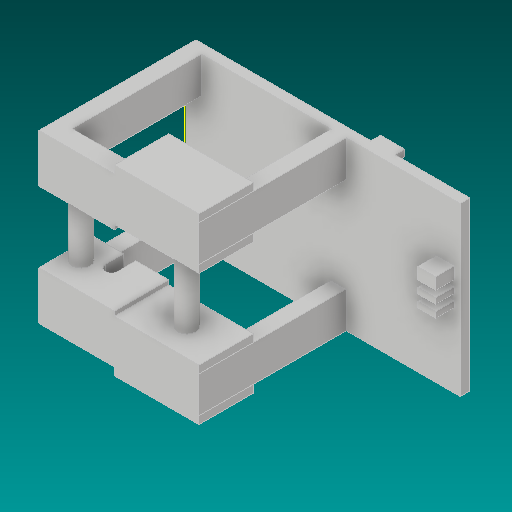
# Autodesk Inventor part: RC_Chassis
Saved by Autodesk Inventor 2019 (Build 230136000, 136)
## iProperties
Created: 2020-12-08
Part Number: RC_Chassis
Material: Generic
Document SubType Name: Modeling
Designer: Jason
Density: 1 g/cm^3
Appearance: Default
Mass: 177.89 g
Surface Area: 666.663 cm^2
Volume: 177.89 cm^3
Author: Jason
Autodesk Inventor part; units mm, degrees
ref_plane "YZ Plane" through (0, 0, 0) normal (1, 0, 0) x (0, 1, 0)
ref_plane "XZ Plane" through (0, 0, 0) normal (0, 1, 0) x (-1, 0, 0)
ref_plane "XY Plane" through (0, 0, 0) normal (0, 0, 1) x (1, 0, 0)
sketch "Sketch1" plane through (0, 0, 0) normal (0, 0, 1) x (1, 0, 0)
  line L0 (0, -53.3468) -> (0, -11.9835) projected
  line L1 (68.5887, -53.3468) -> (0, -53.3468) projected
  line L2 (68.5887, 0) -> (68.5887, -53.3468) projected
  line L3 (0, 0) -> (68.5887, 0) projected
  line L4 (0, -2.1686) -> (0, 0) projected
  line L5 (0, -11.9835) -> (0, -2.1686) projected
  circle A0 centre (15.2894, -50.7921) radius 1.5631 projected
  circle A1 centre (14.0269, -2.6176) radius 1.4996 projected
  line L6 (0, 0) -> (68.5887, 0)
  line L7 (68.5887, 0) -> (68.5887, -53.3468)
  line L8 (68.5887, -53.3468) -> (0, -53.3468)
  line L9 (0, -53.3468) -> (0, 0)
  circle A2 centre (14.0269, -2.6176) radius 1.4996
  circle A3 centre (15.2894, -50.7921) radius 1.5631
  constraints: 8 end point, 2 centre point, 2 coincident, 2 concentric, 2 parallel, 1 horizontal, 1 perpendicular
extrude "Extrusion1" add sketch "Sketch1" against normal blind 5.08 contours A0 | A1
ref_plane "Work Plane1" through (0, 0, 0) normal (0, 0, 1) x (1, 0, 0)
sketch "Sketch2" plane through (0, 0, 0) normal (0, 0, 1) x (1, 0, 0)
  line L0 (0, -53.3468) -> (0, -11.9835) projected
  line L1 (68.5887, 0) -> (68.5887, -53.3468) projected
  line L2 (0, -2.1686) -> (0, 0) projected
  line L3 (0, 0) -> (0, -53.3468)
  line L4 (68.5887, -53.3468) -> (68.5887, 0)
  line L5 (68.5887, -71.3254) -> (144.1005, -71.3254)
  line L6 (144.1005, -71.3254) -> (144.1005, 16.6007)
  line L7 (144.1005, 16.6007) -> (68.5887, 16.6007)
  line L8 (68.5887, 16.6007) -> (68.5887, -71.3254)
  line L9 (68.5887, 16.6007) -> (0, 16.6007)
  line L10 (0, 16.6007) -> (0, 0)
  line L11 (68.5887, -71.3254) -> (0, -71.3254)
  line L12 (0, -71.3254) -> (0, -53.3468)
  constraints: 20 end point, 4 perpendicular, 4 point on line, 3 parallel, 2 horizontal
extrude "Extrusion2" add sketch "Sketch2" along normal mid plane 5.08
sketch "Sketch3" plane through (0, 0, -2.54) normal (0, 0, -1) x (-1, 0, 0)
  line L0 (-125.7496, -4.4471) -> (-125.7496, -55.0115) projected
  line L1 (0, -71.3254) -> (-144.1005, -71.3254) projected
  line L2 (-125.7496, -38.1) -> (-133.2651, -38.1)
  line L3 (-133.2651, -38.1) -> (-133.2651, -17.4625)
  line L4 (-133.2651, -17.4625) -> (-125.7496, -17.4625)
  line L5 (-125.7496, -17.4625) -> (-125.7496, -38.1)
  line L6 (-125.7462, 13.1821) -> (-71.1251, 13.1821)
  line L7 (0, 16.6007) -> (-144.1005, 16.6007) projected
  line L8 (-92.075, 13.1821) -> (-104.775, 13.1821)
  line L9 (-104.775, 13.1821) -> (-104.775, 16.6007)
  line L10 (-104.775, 16.6007) -> (-92.075, 16.6007)
  line L11 (-92.075, 16.6007) -> (-92.075, 13.1821)
  line L12 (-80.6496, -69.3179) -> (-97.3996, -69.3179)
  line L13 (-144.1005, -71.3254) -> (0, -71.3254) projected
  line L14 (-97.3996, -69.3179) -> (-84.496, -69.3179)
  line L15 (-84.496, -69.3179) -> (-84.496, -71.3254)
  line L16 (-84.496, -71.3254) -> (-97.3996, -71.3254)
  line L17 (-97.3996, -71.3254) -> (-97.3996, -69.3179)
  point P0 (0, 0)
  point P1 (-68.5887, -71.3254)
  point P2 (-68.5887, 16.6007)
  constraints: 28 end point, 6 parallel, 4 point on line, 3 horizontal, 3 perpendicular
extrude "Extrusion3" add sketch "Sketch3" along normal blind 5.08
sketch "Sketch9" plane through (0, 0, 2.54) normal (0, 0, 1) x (1, 0, 0)
  line L0 (0, -71.3254) -> (7.9375, -71.3254)
  line L1 (7.9375, -71.3254) -> (7.9375, -52.2754)
  line L2 (7.9375, -52.2754) -> (0, -52.2754)
  line L3 (0, -52.2754) -> (0, -71.3254)
  line L4 (0, 16.6007) -> (7.9502, 16.6007)
  line L5 (7.9502, 16.6007) -> (7.9502, -2.4493)
  line L6 (7.9502, -2.4493) -> (0, -2.4493)
  line L7 (0, -2.4493) -> (0, 16.6007)
  line L8 (76.2, -71.3254) -> (84.1502, -71.3254)
  line L9 (84.1502, -71.3254) -> (84.1502, -52.2754)
  line L10 (84.1502, -52.2754) -> (76.2, -52.2754)
  line L11 (76.2, -52.2754) -> (76.2, -71.3254)
  line L12 (76.2, 16.6007) -> (84.1502, 16.6007)
  line L13 (84.1502, 16.6007) -> (84.1502, -2.4493)
  line L14 (84.1502, -2.4493) -> (76.2, -2.4493)
  line L15 (76.2, -2.4493) -> (76.2, 16.6007)
  line L16 (144.1005, 16.6007) -> (0, 16.6007) projected
  line L17 (0, -71.3254) -> (144.1005, -71.3254) projected
  point P0 (0, 0)
  dimension "d19" = 7.9502
  dimension "d20" = 19.05
  dimension "d21" = 7.9502
  dimension "d22" = 19.05
  dimension "d23" = 7.9502
  dimension "d24" = 19.05
  dimension "d41" = 19.05
  constraints: 32 end point, 8 parallel, 4 horizontal, 4 perpendicular, 2 collinear, 1 point on line
  measures "d19" distance of L5.end L6.end
  measures "d20" distance of L4.end L5.end
  measures "d21" distance of L10.end L9.end
  measures "d22" distance of L9.end L8.end
  measures "d23" distance of L13.end L14.end
  measures "d24" distance of L12.end L13.end
  measures "d41" distance of L0.end L1.end
extrude "Extrusion7" add sketch "Sketch9" along normal blind 67.945
sketch "Sketch10" plane through (0, 0, 2.54) normal (0, 0, 1) x (1, 0, 0)
  line L0 (141.2875, -13.0792) -> (131.7625, -13.0792)
  line L1 (131.7625, -13.0792) -> (131.7625, -19.4292)
  line L2 (131.7625, -19.4292) -> (141.2875, -19.4292)
  line L3 (141.2875, -19.4292) -> (141.2875, -13.0792)
  line L4 (141.2875, -22.6042) -> (131.7625, -22.6042)
  line L5 (131.7625, -22.6042) -> (131.7625, -25.7792)
  line L6 (131.7625, -25.7792) -> (141.2875, -25.7792)
  line L7 (141.2875, -25.7792) -> (141.2875, -22.6042)
  line L8 (141.2875, -28.9542) -> (131.7625, -28.9542)
  line L9 (131.7625, -28.9542) -> (131.7625, -32.1292)
  line L10 (131.7625, -32.1292) -> (141.2875, -32.1292)
  line L11 (141.2875, -32.1292) -> (141.2875, -28.9542)
  line L12 (144.1005, 16.6007) -> (84.1502, 16.6007) projected
  line L13 (84.1502, -71.3254) -> (144.1005, -71.3254) projected
  line L14 (90.4875, -27.3667) -> (109.5375, -27.3667)
  point P0 (0, 0)
  dimension "d30" = 3.175
  dimension "d31" = 3.175
  dimension "d32" = 3.175
  dimension "d33" = 3.175
  dimension "d39" = 6.35
  dimension "d70" = 43.9674
  constraints: 26 end point, 6 parallel, 4 horizontal, 3 perpendicular, 1 point on line, 1 other
  measures "d30" distance of L5.end L4.end
  measures "d31" distance of L9.end L8.end
  measures "d32" distance between parallel lines of L4 L2
  measures "d33" distance between parallel lines of L8 L6
  measures "d39" distance of L0.end L1.end
  measures "d70" distance between parallel lines of L14 L12
extrude "Extrusion8" add sketch "Sketch10" along normal blind 10.16
sketch "Sketch11" plane through (0, 0, 70.485) normal (0, 0, 1) x (1, 0, 0)
  line L0 (0, 16.6007) -> (84.1502, 16.6007)
  line L1 (84.1502, 16.6007) -> (84.1502, -2.4493)
  line L2 (84.1502, -2.4493) -> (0, -2.4493)
  line L3 (0, -2.4493) -> (0, 16.6007)
  line L4 (0, -71.3254) -> (7.9375, -71.3254) projected
  line L5 (0, -71.3254) -> (84.1502, -71.3254)
  line L6 (84.1502, -71.3254) -> (84.1502, -52.2754)
  line L7 (84.1502, -52.2754) -> (0, -52.2754)
  line L8 (0, -52.2754) -> (0, -71.3254)
  point P0 (0, 0)
  dimension "d44" = 19.05
  dimension "d45" = 19.05
  constraints: 16 end point, 4 parallel, 2 horizontal, 2 perpendicular, 1 point on line
  measures "d44" distance between parallel lines of L0 L2
  measures "d45" distance between parallel lines of L5 L7
extrude "Extrusion9" add sketch "Sketch11" along normal blind 9.525
sketch "Sketch12" plane through (0, 0, 70.485) normal (0, 0, -1) x (-1, 0, 0)
  line L0 (0, 16.6007) -> (-92.075, 16.6007) projected
  line L1 (-84.1375, 16.6007) -> (-39.6875, 16.6007)
  line L2 (-39.6875, 16.6007) -> (-39.6875, 20.6375)
  line L3 (-39.6875, 20.6375) -> (-84.1375, 20.6375)
  line L4 (-84.1375, 20.6375) -> (-84.1375, 16.6007)
  line L5 (-84.1375, -6.4861) -> (-39.6875, -6.4861)
  line L6 (-39.6875, -6.4861) -> (-39.6875, -2.4493)
  line L7 (-39.6875, -2.4493) -> (-84.1375, -2.4493)
  line L8 (-84.1375, -2.4493) -> (-84.1375, -6.4861)
  line L9 (-84.1375, -52.2754) -> (-39.6875, -52.2754)
  line L10 (-39.6875, -52.2754) -> (-39.6875, -48.2386)
  line L11 (-39.6875, -48.2386) -> (-84.1375, -48.2386)
  line L12 (-84.1375, -48.2386) -> (-84.1375, -52.2754)
  line L13 (-84.1375, -75.3622) -> (-39.6875, -75.3622)
  line L14 (-39.6875, -75.3622) -> (-39.6875, -71.3254)
  line L15 (-39.6875, -71.3254) -> (-84.1375, -71.3254)
  line L16 (-84.1375, -71.3254) -> (-84.1375, -75.3622)
  line L17 (0, -2.4493) -> (-84.1502, -2.4493) projected
  line L18 (-84.1502, -52.2754) -> (0, -52.2754) projected
  line L19 (0, -71.3254) -> (-84.1502, -71.3254) projected
  line L20 (0, -2.4493) -> (0, -52.2754) projected
  line L21 (-39.6875, -52.2754) -> (0, -52.2754)
  line L22 (0, -52.2754) -> (0, -45.9254)
  line L23 (0, -45.9254) -> (-39.6875, -45.9254)
  line L24 (-39.6875, -45.9254) -> (-39.6875, -52.2754)
  line L25 (-39.6875, -2.4493) -> (0, -2.4493)
  line L26 (0, -2.4493) -> (0, -8.7993)
  line L27 (0, -8.7993) -> (-39.6875, -8.7993)
  line L28 (-39.6875, -8.7993) -> (-39.6875, -2.4493)
  point P0 (0, 0)
  dimension "d46" = 4.0368
  dimension "d53" = 44.45
  dimension "d54" = 6.35
  dimension "d55" = 6.35
  constraints: 48 end point, 12 collinear, 12 parallel, 6 horizontal, 6 perpendicular, 3 point on line
  measures "d46" distance of L3.end L1.start
  measures "d53" distance of L2.end L3.end
  measures "d54" distance of L22.end L21.end
  measures "d55" distance of L25.end L26.end
extrude "Extrusion10" add sketch "Sketch12" along normal blind 19.05 and the other way blind 9.525
sketch "Sketch13" plane through (0, -45.9254, 51.435) normal (0, 1, 0) x (1, 0, 0)
  line L0 (19.1249, 12.586) -> (19.1249, -9.639) construction
  line L1 (15.9499, 12.586) -> (15.9499, -9.639)
  line L2 (22.2999, -9.639) -> (22.2999, 12.586)
  arc A0 (22.2999, 12.586) -> (15.9499, 12.586) centre (19.1249, 12.586) ccw
  arc A1 (15.9499, -9.639) -> (22.2999, -9.639) centre (19.1249, -9.639) ccw
  point P0 (0, 51.435)
  point P1 (19.1249, 1.4735)
  constraints: 8 end point, 4 point on circle, 4 tangent, 2 centre point, 1 midpoint, 1 parallel, 1 vertical
extrude "Extrusion11" cut sketch "Sketch13" against normal blind 8.255
sketch "Sketch14" plane through (0, -8.7993, 51.435) normal (0, -1, 0) x (1, 0, 0)
  line L0 (19.1249, 12.586) -> (19.1249, -9.639) construction
  line L1 (15.9499, 12.586) -> (15.9499, -9.639)
  line L2 (22.2999, -9.639) -> (22.2999, 12.586)
  arc A0 (22.2999, 12.586) -> (15.9499, 12.586) centre (19.1249, 12.586) ccw
  arc A1 (15.9499, -9.639) -> (22.2999, -9.639) centre (19.1249, -9.639) ccw
  point P0 (0, 51.435)
  point P1 (19.1249, 1.4735)
  constraints: 8 end point, 4 point on circle, 4 tangent, 2 centre point, 1 midpoint, 1 parallel, 1 vertical
extrude "Extrusion12" cut sketch "Sketch14" against normal blind 8.255
sketch "Sketch15" plane through (39.6875, -6.4861, 51.435) normal (0, -1, 0) x (1, 0, 0)
  circle A0 centre (23.8125, 14.2875) radius 4.7625
  line L0 (-31.7373, -48.895) -> (-31.7373, 19.05) projected
  circle A1 centre (-31.7373, 14.2875) radius 4.7625
  point P0 (-39.6875, -51.435)
  dimension "d64" = 9.525
  constraints: 2 centre point, 1 point on line
  measures "d64" diameter of A1
extrude "Extrusion13" add sketch "Sketch15" along normal blind 44.45
body "Solid1"
